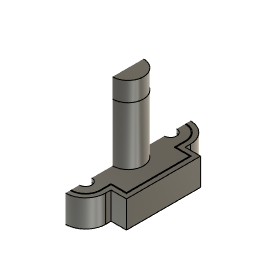
light-thing (Autodesk Fusion 360 design; units mm, degrees)
Autodesk Fusion 360 part; units mm, degrees
sketch "Skizze1" plane through (0, 0, 0) normal (0, 0, 1) x (1, 0, 0)
  line L0 (8, 15) -> (-8, 15)
  line L1 (-8, 15) -> (-8, -15)
  line L2 (-8, -15) -> (8, -15)
  line L3 (8, -15) -> (8, 15)
  line L4 (8, 15) -> (-8, -15) construction
  line L5 (-8, 15) -> (8, -15) construction
  line L6 (-8, 7) -> (8, 7)
  line L7 (-8, -7) -> (8, -7)
  line L8 (6.6, -13.6) -> (6.6, 13.6)
  line L9 (6.6, 13.6) -> (-6.6, 13.6)
  line L10 (-6.6, 13.6) -> (-6.6, -13.6)
  line L11 (-6.6, -13.6) -> (6.6, -13.6)
  line L12 (8, -7) -> (8, -15)
  circle A0 centre (0, -11) radius 1.6
  line L13 (8, 15) -> (8, 7)
  circle A1 centre (0, 11) radius 1.6
  line L14 (-4, 0) -> (4, 0)
  line L15 (4, 0) -> (4, -4)
  line L16 (4, -4) -> (-4, -4)
  line L17 (-4, -4) -> (-4, 0)
  circle A2 centre (0, 11) radius 4
  circle A3 centre (0, -11) radius 4
  line L18 (-4, 11) -> (4, 11)
  line L19 (4, 11) -> (4, 7)
  line L20 (4, 7) -> (-4, 7)
  line L21 (-4, 7) -> (-4, 11)
  line L22 (-4, -11) -> (4, -11)
  line L23 (4, -11) -> (4, -7)
  line L24 (4, -7) -> (-4, -7)
  line L25 (-4, -7) -> (-4, -11)
  line L26 (-8, -8.4) -> (8, -8.4)
  line L27 (-8, 8.4) -> (8, 8.4)
  point P0 (8, -11)
  point P1 (8, 11)
  dimension "d1" = 16
  dimension "d2" = 30
  dimension "d3" = 8
  dimension "d4" = 8
  dimension "d5" = -1.4
  dimension "d6" = 3.2
  dimension "d7" = 3.2
  dimension "d8" = 8
  dimension "d9" = 4
  dimension "d14" = 8
  dimension "d15" = 8
  dimension "d16" = 8
  dimension "d17" = 8
  dimension "d18" = 1.4
  dimension "d19" = 1.4
  constraint horizontal L0
  constraint perpendicular L0 L1
  constraint parallel L0 L2
  constraint parallel L1 L3
  constraint coincident L4 origin
  constraint coincident L5 origin
  constraint coincident L1 L6.start
  constraint coincident L3 L6.end
  constraint perpendicular L3 L6
  constraint coincident L1 L7.start
  constraint coincident L3 L7.end
  constraint perpendicular L3 L7
  constraint midpoint L12 P0
  constraint midpoint L13 P1
  constraint horizontal L14
  constraint vertical L15
  constraint horizontal L16
  constraint vertical L17
  constraint concentric A1 A2
  constraint concentric A0 A3
  constraint horizontal L18
  constraint vertical L19
  constraint horizontal L20
  constraint vertical L21
  constraint coincident A2 L18.start
  constraint horizontal L22
  constraint vertical L23
  constraint horizontal L24
  constraint vertical L25
  constraint coincident A3 L22.start
  constraint coincident L1 L26.start
  constraint perpendicular L8 L26
  constraint coincident L1 L27.start
  constraint coincident L13 L27.end
  constraint perpendicular L13 L27
  measures "d1" distance of L1.end L2.end
  measures "d2" distance of L0.end L1.end
  measures "d3" distance of L0 L6
  measures "d4" distance of L2 L7
  measures "d6" diameter of A0
  measures "d7" diameter of A1
  measures "d8" distance of L14.start L14.end
  measures "d9" distance of L14.start L16.end
  measures "d14" diameter of A2
  measures "d15" diameter of A3
  measures "d16" distance of L18.start L18.end
  measures "d17" distance of L22.start L22.end
  measures "d18" distance of L7 L26
  measures "d19" distance of L6 L27
extrude "Extrusion1" add sketch "Skizze1" along normal blind 2 contours L9 A2 | L3 L6 L8 L13 L27 | L9 A1 A2 L18 | L3 L6 L7 L8 | L6 L8 L19 L27 | L1 L6 L10 L27 | A2 L19 L27 | A1 A2 L18 L27 | A2 L21 L27 | L3 L7 L8 L12 L26 | L6 L7 L8 L10 L20 L24 | L6 A2 L19 L20 L27 | L1 L6 L7 L10 | L6 L10 L21 L27 | A2 L27 | L6 A2 L20 L21 L27 | L7 L8 L23 L26 | L1 L7 L10 L26 | L7 A3 L23 L24 L26 | L7 L10 L25 L26 | L11 A3 | A3 L23 L26 | L7 A3 L24 L25 L26 | A3 L26 | L11 A0 A3 L22 | A0 A3 L22 L26 | A3 L25 L26 makes body 1
sketch "Skizze2" plane through (0, 0, 2) normal (0, 0, 1) x (-1, 0, 0)
  line L0 (-4, 4) -> (4, 4)
  line L1 (4, 4) -> (4, 0)
  line L2 (4, 0) -> (-4, 0)
  line L3 (-4, 0) -> (-4, 4)
  circle A0 centre (0, 11) radius 1.6
  circle A1 centre (0, -11) radius 1.6
  line L4 (8, -8.4) -> (8, 8.4)
  line L5 (-8, 8.4) -> (-8, -8.4)
  line L6 (8, -7) -> (-8, -7)
  line L7 (8, -15) -> (8, 15)
  line L8 (8, 7) -> (-8, 7)
  line L9 (6.6, -13.6) -> (6.6, 13.6)
  line L10 (-6.6, 13.6) -> (-6.6, -13.6)
  line L11 (4, 8.4) -> (4, 11)
  arc A2 (4, 11) -> (-4, 11) centre (0, 11) ccw
  line L12 (-4, 11) -> (-4, 8.4)
  line L13 (-4, -8.4) -> (-4, -11)
  arc A3 (-4, -11) -> (4, -11) centre (0, -11) ccw
  line L14 (4, -11) -> (4, -8.4)
  line L15 (8, 8.4) -> (4, 8.4)
  line L16 (-4, 8.4) -> (-8, 8.4)
  line L17 (-8, -8.4) -> (-4, -8.4)
  line L18 (4, -8.4) -> (8, -8.4)
extrude "Extrusion2" add sketch "Skizze2" along normal blind 4 contours L4 L6 L7 L9 L18 | L4 L6 L7 L8 L9 | L6 L9 L10 L13 A3 L14 L17 L18 | L4 L7 L8 L9 L15 | L8 L9 L10 L11 A2 L12 L15 L16 | L5 L6 L10 L17 | L5 L6 L8 L10 | L5 L8 L10 L16 bodies 1
sketch "Skizze3" plane through (0, 0, 6) normal (0, 0, 1) x (-1, 0, 0)
  line L0 (6.6, 7) -> (6.6, -7)
  line L1 (6.6, -7) -> (-6.6, -7)
  line L2 (-6.6, -7) -> (-6.6, 7)
  line L3 (-6.6, 7) -> (6.6, 7)
  circle A0 centre (0, -11) radius 1.6
  circle A1 centre (0, 11) radius 1.6
  line L4 (4, -8.4) -> (8, -8.4)
  line L5 (8, -8.4) -> (8, 8.4)
  line L6 (8, 8.4) -> (4, 8.4)
  line L7 (4, 8.4) -> (4, 11)
  arc A2 (4, 11) -> (-4, 11) centre (0, 11) ccw
  line L8 (-4, 11) -> (-4, 8.4)
  line L9 (-4, 8.4) -> (-8, 8.4)
  line L10 (-8, 8.4) -> (-8, -8.4)
  line L11 (-8, -8.4) -> (-4, -8.4)
  line L12 (-4, -8.4) -> (-4, -11)
  arc A3 (-4, -11) -> (4, -11) centre (0, -11) ccw
  line L13 (4, -11) -> (4, -8.4)
  circle A4 centre (0, 0) radius 3.2
  line L14 (-3.8, -8.2) -> (-3.8, -11)
  arc A5 (-3.8, -11) -> (3.8, -11) centre (0, -11) ccw
  line L15 (3.8, -11) -> (3.8, -8.2)
  line L16 (3.8, -8.2) -> (7.8, -8.2)
  line L17 (7.8, -8.2) -> (7.8, 8.2)
  line L18 (7.8, 8.2) -> (3.8, 8.2)
  line L19 (3.8, 8.2) -> (3.8, 11)
  arc A6 (3.8, 11) -> (-3.8, 11) centre (0, 11) ccw
  line L20 (-3.8, 11) -> (-3.8, 8.2)
  line L21 (-3.8, 8.2) -> (-7.8, 8.2)
  line L22 (-7.8, 8.2) -> (-7.8, -8.2)
  line L23 (-7.8, -8.2) -> (-3.8, -8.2)
  dimension "d20" = 6.4
  dimension "d35" = -0.2
  constraint coincident A4.centre origin
  measures "d20" diameter of A4
extrude "Extrusion3" add sketch "Skizze3" along normal blind 1 separate body contours L0 L1 L2 L3 | L14 A5 L15 L16 L17 L18 L19 A6 L20 L21 L22 L23 makes body 2
sketch "Skizze4" plane through (0, 0, 7) normal (0, 0, 1) x (-1, 0, 0)
  circle A0 centre (0, 0) radius 3.2
  circle A1 centre (0, 11) radius 1.6
  circle A2 centre (0, -11) radius 1.6
  circle A3 centre (0, 0) radius 3.2
  circle A4 centre (0, 0) radius 4
  line L0 (-7.8, -8.2) -> (-3.8, -8.2)
  line L1 (-3.8, -8.2) -> (-3.8, -11)
  arc A5 (-3.8, -11) -> (3.8, -11) centre (0, -11) ccw
  line L2 (3.8, -11) -> (3.8, -8.2)
  line L3 (3.8, -8.2) -> (7.8, -8.2)
  line L4 (7.8, -8.2) -> (7.8, 8.2)
  line L5 (7.8, 8.2) -> (3.8, 8.2)
  line L6 (3.8, 8.2) -> (3.8, 11)
  arc A6 (3.8, 11) -> (-3.8, 11) centre (0, 11) ccw
  line L7 (-3.8, 11) -> (-3.8, 8.2)
  line L8 (-3.8, 8.2) -> (-7.8, 8.2)
  line L9 (-7.8, 8.2) -> (-7.8, -8.2)
  dimension "d23" = 8
  constraint coincident A0.centre A3.centre
  measures "d23" diameter of A4
extrude "Extrusion4" add sketch "Skizze4" along normal blind 18 contours A4 bodies 2
sketch "Skizze15" plane through (0, 0, 25) normal (0, 0, 1) x (-1, 0, 0)
  circle A0 centre (0, 0) radius 3.2
  circle A1 centre (0, 0) radius 4
  circle A2 centre (0, 0) radius 4
  circle A3 centre (0, 0) radius 3.2
  circle A4 centre (0, 0) radius 2.6
  circle A5 centre (0, 0) radius 3.1
  dimension "d39" = -0.6
  dimension "d40" = -0.1
extrude "Extrusion7" add sketch "Skizze15" along normal blind 2 contours A0 A3 | A1 A2 | A4 | A5 bodies 2
ref_plane "Arbeitsebene3" through (0, 0, 22) normal (0, 0, 1) x (-1, 0, 0)
split "Teilen1" by plane through (0, 0, 22) normal (0, 0, 1) bodies 2 makes body 3 at (-3.9801, -0.3983, 23.6667)
extrude "Extrusion8" add sketch "Skizze15" against normal blind 8 contours A5 bodies 3
extrude "Extrusion9" add sketch "Skizze15" against normal blind 3 contours A0 A3 bodies 3
ref_plane "Arbeitsebene2" through (0, 0, 3) normal (-1, 0, 0) x (0, -1, 0)
sketch "Skizze9" plane through (0, 0, 0) normal (0, 0, -1) x (1, 0, 0)
  circle A0 centre (0, -11) radius 1.6
  line L0 (-4, 4) -> (4, 4)
  line L1 (4, 4) -> (4, 0)
  line L2 (4, 0) -> (-4, 0)
  line L3 (-4, 0) -> (-4, 4)
  circle A1 centre (0, 11) radius 1.6
  line L4 (-4, 8.4) -> (-8, 8.4)
  line L5 (-8, 8.4) -> (-8, -8.4)
  line L6 (-8, -8.4) -> (-4, -8.4)
  line L7 (-4, -8.4) -> (-4, -11)
  arc A2 (-4, -11) -> (4, -11) centre (0, -11) ccw
  line L8 (4, -11) -> (4, -8.4)
  line L9 (4, -8.4) -> (8, -8.4)
  line L10 (8, -8.4) -> (8, 8.4)
  line L11 (8, 8.4) -> (4, 8.4)
  line L12 (4, 8.4) -> (4, 11)
  arc A3 (4, 11) -> (-4, 11) centre (0, 11) ccw
  line L13 (-4, 11) -> (-4, 8.4)
  line L14 (5.2, 9.6) -> (5.2, 11)
  arc A4 (5.2, 11) -> (-5.2, 11) centre (0, 11) ccw
  line L15 (-5.2, 11) -> (-5.2, 9.6)
  line L16 (-5.2, 9.6) -> (-9.2, 9.6)
  line L17 (-9.2, 9.6) -> (-9.2, -9.6)
  line L18 (-9.2, -9.6) -> (-5.2, -9.6)
  line L19 (-5.2, -9.6) -> (-5.2, -11)
  arc A5 (-5.2, -11) -> (5.2, -11) centre (0, -11) ccw
  line L20 (5.2, -11) -> (5.2, -9.6)
  line L21 (5.2, -9.6) -> (9.2, -9.6)
  line L22 (9.2, -9.6) -> (9.2, 9.6)
  line L23 (9.2, 9.6) -> (5.2, 9.6)
  dimension "d32" = 1.2
extrude "Extrusion6" add sketch "Skizze9" against normal blind 7 separate body contours L14 A4 L15 L16 L17 L18 L19 A5 L20 L21 L22 L23 makes body 4
combine "Kombinieren1" operation add target body 1 tool bodies 4
ref_plane "Arbeitsebene4" through (0, 0, 26.6) normal (0, 0, 1) x (-1, 0, 0)
sketch "Skizze16" plane through (0, 0, 26.6) normal (0, 0, 1) x (1, 0, 0)
  circle A0 centre (0, 0) radius 4
  circle A1 centre (0, 0) radius 3.6
  dimension "d46" = -0.4
extrude "Extrusion10" cut sketch "Skizze15" along normal blind 0.5 contours A4 bodies 3
equation "d4 = d3"
